Autodesk Inventor part; units mm, degrees
(part 16 of 16)
sketch "Sketch9" plane through (0, 0, 0) normal (1, 0, 0) x (0, 1, 0)
  line L0 (133.6268, 0) -> (133.5377, 0) projected
  line L1 (133.6268, 0) -> (133.6268, 39.6875) projected
  line L2 (133.6268, 39.6875) -> (133.5377, 39.6875) projected
  line L3 (133.5377, 0) -> (133.5377, 39.6875) projected
  line L4 (99.4446, 0) -> (133.6268, 0) projected
  line L5 (99.4446, 0) -> (99.4446, 39.6875) projected
  line L6 (99.4446, 39.6875) -> (133.6268, 39.6875) projected
  line L7 (133.6268, 0) -> (133.6268, 39.6875) projected
  line L8 (133.6268, 0) -> (133.5377, 0) projected
  line L9 (133.6268, 0) -> (133.6268, 39.6875) projected
  line L10 (133.6268, 39.6875) -> (133.5377, 39.6875) projected
  line L11 (133.5377, 0) -> (133.5377, 39.6875) projected
  line L12 (141.8739, 0) -> (141.8739, 39.6875) projected
  line L13 (133.5377, 39.6875) -> (141.8739, 39.6875) projected
  line L14 (141.8739, 0) -> (106.8377, 39.6875)
  line L15 (133.5377, 39.6875) -> (99.4446, 39.6875) projected
  line L16 (141.8739, 0) -> (141.8739, 39.6875)
  line L17 (141.8739, 39.6875) -> (106.8377, 39.6875)
  point P0 (0, 0)
  constraints: 6 end point, 2 collinear, 1 point on line
extrude "Extrusion7" cut sketch "Sketch9" along normal through all both and the other way through all contours L14 L3 L2 L1 | L1 L13 L12 L14 | L14 L6 L3
sketch "Sketch10" plane through (0, 0, 0) normal (1, 0, 0) x (0, 1, 0)
  line L0 (133.6268, 9.3419) -> (141.8739, 0) projected
  line L1 (106.8377, 39.6875) -> (133.6268, 9.3419) projected
  line L2 (97.1696, 39.6875) -> (106.6946, 39.6875) projected
  line L3 (141.8739, 0) -> (106.6946, 39.6875)
  line L4 (106.6946, 39.6875) -> (108.816, 39.6875)
  line L5 (108.816, 39.6875) -> (143.9953, 0)
  line L6 (143.9953, 0) -> (141.8739, 0)
  point P0 (0, 0)
  dimension "d29" = 1.5875
  constraints: 8 end point, 2 parallel, 1 horizontal
  measures "d29" distance between parallel lines of L3 L5
extrude "Extrusion8" add sketch "Sketch10" along normal mid plane 127
sketch "Sketch11" plane through (0, 0, 39.6875) normal (0, 0, 1) x (1, 0, 0)
  line L0 (-34.8862, 132.3193) -> (-58.5344, 108.1018) projected
  arc A0 (34.9717, 132.2316) -> (-34.8862, 132.3193) centre (-0.0477, 60.1323) ccw projected
  line L1 (58.5338, 108.1018) -> (34.9717, 132.2316) projected
  line L2 (-69.207, 99.4446) -> (-62.1273, 106.6946) projected
  line L3 (-62.1273, 106.6946) -> (-35.8282, 133.6268) projected
  arc A1 (-0.0477, 141.8739) -> (-35.8282, 133.6268) centre (-0.0477, 60.1323) ccw projected
  arc A2 (35.9152, 133.5377) -> (-0.0477, 141.8739) centre (-0.0477, 60.1323) ccw projected
  line L4 (35.9152, 133.5377) -> (62.1266, 106.6946) projected
  line L5 (-62.1273, 106.6946) -> (-63.5, 106.6946) projected
  line L6 (-62.1273, 106.6946) -> (-63.5, 106.6946)
  line L7 (-63.5, 106.6946) -> (-63.5, 141.8739) projected
  line L8 (-63.5, 106.6946) -> (-63.5, 141.8739)
  line L9 (-63.5, 141.8739) -> (-63.5, 143.9953) projected
  line L10 (-63.5, 143.9403) -> (-63.5, 141.8739)
  line L11 (63.5, 143.9953) -> (-63.5, 143.9953) projected
  line L12 (-63.5, 143.9953) -> (0, 143.9953)
  line L13 (63.5, 143.9953) -> (63.5, 141.8739) projected
  line L14 (0, 143.9953) -> (63.5, 143.9953)
  line L15 (63.5, 143.9953) -> (63.5, 106.6946)
  line L16 (62.1266, 106.6946) -> (69.2061, 99.4446) projected
  line L17 (63.5, 106.6946) -> (62.1266, 106.6946)
  point P0 (0, 0)
  constraints: 14 end point, 3 perpendicular, 2 horizontal, 1 collinear, 1 midpoint
extrude "Extrusion9" cut sketch "Sketch11" against normal through all
extrude "Extrusion10" cut sketch "Sketch3" against normal through all contours A5 | A7 A8 A9 A10 A11 A6 | A12 | A14 A15 A16 A17 A18 A13 | A19 | A21 A22 A23 A24 A25 A20 | A26 | A28 A29 A30 A31 A32 A27 | A33 | A34 | A35 | A36
ref_plane "Work Plane2" through (0, 0, 34.29) normal (0, 0, -1) x (-1, 0, 0)
sketch "Sketch13" plane through (0, 0, 34.29) normal (0, 0, -1) x (-1, 0, 0)
  circle A0 centre (-45.7832, 101.9321) radius 4.7625 projected
  arc A1 (-43.5737, 46.9132) -> (-47.9928, 46.9132) centre (-45.7832, 51.1321) ccw projected
  line L0 (-43.5737, 46.9132) -> (43.5737, 46.9132) projected
  arc A2 (47.9928, 46.9132) -> (43.5737, 46.9132) centre (45.7832, 51.1321) ccw projected
  line L1 (47.9928, 46.9132) -> (53.9435, 46.9132) projected
  arc A3 (53.9435, 46.9132) -> (67.6381, 98.779) centre (-28.0956, 96.3156) ccw projected
  line L2 (67.6381, 98.779) -> (58.5344, 108.1018) projected
  line L3 (58.5344, 108.1018) -> (-58.5338, 108.1018) projected
  line L4 (-58.5338, 108.1018) -> (-67.638, 98.7782) projected
  arc A4 (-67.638, 98.7782) -> (-54.02, 46.9132) centre (28.0925, 96.1937) ccw projected
  line L5 (-54.02, 46.9132) -> (-47.9928, 46.9132) projected
  circle A5 centre (45.7832, 101.9321) radius 4.7625 projected
  circle A6 centre (-45.7832, 101.9321) radius 4.7625 projected
  arc A7 (47.9928, 46.9132) -> (43.5737, 46.9132) centre (45.7832, 51.1321) ccw projected
  circle A8 centre (45.7832, 101.9321) radius 4.7625 projected
  circle A9 centre (-45.7832, 101.9321) radius 4.7625
  circle A10 centre (-45.7832, 101.9321) radius 7.0485
  circle A11 centre (-45.7832, 51.1321) radius 7.0485
  circle A12 centre (-45.7832, 51.1321) radius 4.7625
  circle A13 centre (45.7832, 51.1321) radius 4.7625
  circle A14 centre (45.7832, 51.1321) radius 7.0485
  circle A15 centre (45.7832, 101.9321) radius 7.0485
  circle A16 centre (45.7832, 101.9321) radius 4.7625
  point P0 (0, 0)
  dimension "d37" = 2.286
  constraints: 8 centre point, 7 coincident, 6 equal radius, 1 concentric
  measures "d37" radial gap between concentric circles of A15 A5
extrude "Extrusion11" add sketch "Sketch13" against normal up to next contours A1 L5 A11 L0 | L0 A11 L5 A12 | A14 L1 A2 L0 | L0 A13 L1 A14 | A10 L3 | L3 A10 | A15 L3 | L3 A15
sketch "Sketch14" plane through (-69.207, 99.4446, 0) normal (-0.7154653, 0.6986483, 0) x (0, 0, 1)
  line L0 (0, 167.0871) -> (0, -112.8454) projected
  line L1 (0, 47.7762) -> (11.6972, 47.7762) projected
  point P0 (0, -22.7978)
  point P1 (9.525, 35.0762)
  dimension "d40" = 9.525
  dimension "d41" = 12.7
  measures "d40" distance from line of L0 point (9.525, 35.076)
  measures "d41" distance from line of point (9.525, 35.076) L1
hole "Hole1" at (-44.701, 124.5404, 9.525) direction (0.7154653, -0.6986483, 0) diameter 6.35 depth 12.7 tip angle 118
mirror "Mirror1" about plane through (0, 0, 0) normal (1, 0, 0) of "Hole1"
sketch "Sketch15" plane through (0, 0, 0) normal (1, 0, 0) x (0, 1, 0)
  circle A0 centre (49.5446, 9.525) radius 3.175
  ellipse E0 centre (124.5404, 9.525) end of major axis (124.5404, 12.7) minor radius 2.2716 projected
  line L0 (46.3457, 39.6875) -> (99.4446, 39.6875) projected
  line L1 (46.3696, 39.6875) -> (46.3696, 34.29) projected
  point P0 (0, 0)
  dimension "d49" = 6.35
  dimension "d50" = 3.175
  constraints: 1 centre point, 1 horizontal alignment, 1 other
  measures "d49" diameter of A0
  measures "d50" distance from line of L1 A0.centre
extrude "Extrusion12" cut sketch "Sketch15" along normal through all both and the other way through all contours A0
sketch "Sketch16" plane through (0, 0, 0) normal (0, 1, 0) x (-1, 0, 0)
  line L0 (-19.05, -6.1946) -> (19.05, -6.1946)
  line L1 (19.05, -6.1946) -> (19.05, 4.7625)
  line L2 (19.05, 4.7625) -> (-19.05, 4.7625)
  line L3 (-19.05, 4.7625) -> (-19.05, -6.1946)
  line L4 (-45.8908, 0) -> (-0.0538, 0) projected
  point P0 (0, 0)
  point P1 (0, -6.1946)
  dimension "d53" = 4.7625
  dimension "d54" = 38.1
  constraints: 8 end point, 2 parallel, 1 horizontal, 1 midpoint, 1 perpendicular, 1 vertical alignment
  measures "d53" distance between parallel lines of L4 L2
  measures "d54" distance of L0.start L0.end
extrude "Extrusion13" cut sketch "Sketch16" along normal blind 25.4
sketch "Sketch17" plane through (-60.0558, 108.816, 39.6875) normal (0, 0.7483314, 0.6633251) x (1, 0, 0)
  line L0 (53.1651, 39.4078) -> (64.8681, 39.4078) construction
  line L1 (64.8681, 39.4078) -> (64.8681, 33.1834) construction
  line L2 (64.8681, 33.1834) -> (53.1651, 33.1834) construction
  line L3 (53.1651, 33.1834) -> (53.1651, 39.4078) construction
  spline S0 degree 2 poles (56.2625, 33.1834) (55.0324, 33.1834) (53.7085, 34.369) (53.7085, 35.5151) knots 0 0 0 1 2 2 2
  line L4 (53.7085, 35.5151) -> (53.7085, 39.4078)
  line L5 (53.7085, 39.4078) -> (55.2399, 39.4078)
  line L6 (55.2399, 39.4078) -> (55.2399, 35.604)
  spline S1 degree 2 poles (55.2399, 35.604) (55.2399, 34.9668) (55.7191, 34.3443) (56.2625, 34.3443) knots 0 0 0 1 2 2 2
  spline S2 degree 2 poles (56.2625, 34.3443) (56.7911, 34.3443) (57.2851, 34.9421) (57.2851, 35.604) knots 0 0 0 1 2 2 2
  line L7 (57.2851, 35.604) -> (57.2851, 39.4078)
  line L8 (57.2851, 39.4078) -> (58.8165, 39.4078)
  line L9 (58.8165, 39.4078) -> (58.8165, 35.52)
  spline S3 degree 2 poles (58.8165, 35.52) (58.8165, 34.3937) (57.5272, 33.1834) (56.2625, 33.1834) knots 0 0 0 1 2 2 2
  spline S4 degree 2 poles (64.6803, 37.4862) (64.6803, 37.0613) (64.4086, 36.2907) (64.1567, 36.0338) knots 0 0 0 1 2 2 2
  spline S5 degree 2 poles (64.1567, 36.0338) (64.0035, 35.8708) (63.6281, 35.604) (63.4058, 35.5102) knots 0 0 0 1 2 2 2
  spline S6 degree 2 poles (63.4058, 35.5102) (63.1786, 35.4163) (62.65, 35.3076) (62.3239, 35.3076) knots 0 0 0 1 2 2 2
  line L10 (62.3239, 35.3076) -> (61.5237, 35.3076)
  line L11 (61.5237, 35.3076) -> (61.5237, 33.3118)
  line L12 (61.5237, 33.3118) -> (59.9922, 33.3118)
  line L13 (59.9922, 33.3118) -> (59.9922, 39.4078)
  line L14 (59.9922, 39.4078) -> (62.3585, 39.4078)
  spline S7 degree 2 poles (62.3585, 39.4078) (62.8822, 39.4078) (63.6479, 39.2152) (63.9591, 39.0077) knots 0 0 0 1 2 2 2
  spline S8 degree 2 poles (63.9591, 39.0077) (64.3049, 38.7755) (64.6803, 38.0148) (64.6803, 37.4862) knots 0 0 0 1 2 2 2
  spline S9 degree 2 poles (63.1094, 37.4466) (63.1094, 37.7085) (62.8624, 38.079) (62.6944, 38.1481) knots 0 0 0 1 2 2 2
  spline S10 degree 2 poles (62.6944, 38.1481) (62.4771, 38.242) (62.0819, 38.2716) (61.741, 38.2716) knots 0 0 0 1 2 2 2
  line L15 (61.741, 38.2716) -> (61.5237, 38.2716)
  line L16 (61.5237, 38.2716) -> (61.5237, 36.4438)
  line L17 (61.5237, 36.4438) -> (61.6323, 36.4438)
  spline S11 degree 2 poles (61.6323, 36.4438) (61.8448, 36.4438) (62.2301, 36.4537) (62.3733, 36.4784) knots 0 0 0 1 2 2 2
  spline S12 degree 2 poles (62.3733, 36.4784) (62.4968, 36.4982) (62.7685, 36.6167) (62.8426, 36.6908) knots 0 0 0 1 2 2 2
  spline S13 degree 2 poles (62.8426, 36.6908) (63.0007, 36.839) (63.1094, 37.17) (63.1094, 37.4466) knots 0 0 0 1 2 2 2
  point P0 (60.0558, -42.481)
  constraints: 2 other
extrude "Extrusion14" add sketch "Sketch17" along normal blind 1.27
equation "\"d3\" = d2"
equation "\"d14\" = d15"
equation "\"d15\" = d13"
equation "\"d18\" = d14"
body "Solid1"
